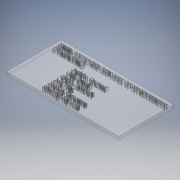
# Autodesk Inventor part: Group Name Plate
Saved by Autodesk Inventor 2018 (Build 220112000, 112)
## iProperties
Created: 2018-11-06
Part Number: Group Name Plate
Material: Generic
Document SubType Name: Modeling
Designer: P300023
Density: 1 g/cm^3
Appearance: Polycarbonate - Clear
Author: P300023
Autodesk Inventor part; units mm, degrees
(part 1 of 4)
ref_plane "YZ Plane" through (0, 0, 0) normal (1, 0, 0) x (0, 1, 0)
ref_plane "XZ Plane" through (0, 0, 0) normal (0, 1, 0) x (-1, 0, 0)
ref_plane "XY Plane" through (0, 0, 0) normal (0, 0, 1) x (1, 0, 0)
sketch "Sketch1" plane through (0, 0, 0) normal (0, 0, 1) x (1, 0, 0)
  line L0 (0, 0) -> (-100, 0)
  line L1 (-100, 0) -> (-100, -49.027)
  line L2 (-100, -49.027) -> (0, -49.027)
  line L3 (0, -49.027) -> (0, 0)
  dimension "d0" = 100
  dimension "d1" = 49.027
  constraints: 8 end point, 2 parallel, 1 horizontal, 1 perpendicular
  measures "d0" distance of L2.end L1.end
  measures "d1" distance of L1.end L0.end
extrude "Extrusion1" add sketch "Sketch1" along normal blind 3
sketch "Sketch2" plane through (0, 0, 3) normal (0, 0, 1) x (1, 0, 0)
  line L0 (-72.5, -15.3818) -> (-27.5, -15.3818) construction
  line L1 (-27.5, -15.3818) -> (-27.5, -49.5595) construction
  line L2 (-27.5, -49.5595) -> (-72.5, -49.5595) construction
  line L3 (-72.5, -49.5595) -> (-72.5, -15.3818) construction
  line L4 (0, 0) -> (-100, 0) projected
  line L5 (-100, -49.027) -> (0, -49.027) projected
  line L6 (0, -49.027) -> (0, 0) projected
  line L7 (-97.5, -2.505) -> (-2.5, -2.505) construction
  line L8 (-2.5, -2.505) -> (-2.5, -5.8685) construction
  line L9 (-2.5, -5.8685) -> (-97.5, -5.8685) construction
  line L10 (-97.5, -5.8685) -> (-97.5, -2.505) construction
  line L11 (-100, 0) -> (-100, -49.027) projected
  spline S0 degree 2 poles (-70.97, -17.892) (-70.97, -18.3121) (-71.4835, -18.7685) (-71.9165, -18.7685) knots 0 0 0 1 2 2 2
  spline S1 degree 2 poles (-71.9165, -18.7685) (-72.0203, -18.7685) (-72.3652, -18.7322) (-72.4818, -18.7063) knots 0 0 0 1 2 2 2
  line L12 (-72.4818, -18.7063) -> (-72.4818, -18.2966)
  line L13 (-72.4818, -18.2966) -> (-72.4585, -18.2966)
  spline S2 degree 2 poles (-72.4585, -18.2966) (-72.3703, -18.3277) (-72.1084, -18.4003) (-71.9736, -18.4003) knots 0 0 0 1 2 2 2
  spline S3 degree 2 poles (-71.9736, -18.4003) (-71.7765, -18.4003) (-71.5405, -18.3096) (-71.4861, -18.2266) knots 0 0 0 1 2 2 2
  spline S4 degree 2 poles (-71.4861, -18.2266) (-71.4264, -18.141) (-71.3953, -17.892) (-71.3953, -17.7287) knots 0 0 0 1 2 2 2
  line L14 (-71.3953, -17.7287) -> (-71.3953, -15.8642)
  line L15 (-71.3953, -15.8642) -> (-72.0721, -15.8642)
  line L16 (-72.0721, -15.8642) -> (-72.0721, -15.5245)
  line L17 (-72.0721, -15.5245) -> (-70.97, -15.5245)
  line L18 (-70.97, -15.5245) -> (-70.97, -17.892)
  spline S5 degree 2 poles (-69.3311, -18.7789) (-69.9068, -18.7789) (-70.5395, -18.1332) (-70.5395, -17.5368) knots 0 0 0 1 2 2 2
  spline S6 degree 2 poles (-70.5395, -17.5368) (-70.5395, -16.9507) (-69.925, -16.2557) (-69.4297, -16.2557) knots 0 0 0 1 2 2 2
  spline S7 degree 2 poles (-69.4297, -16.2557) (-69.2066, -16.2557) (-68.8618, -16.3854) (-68.7347, -16.5228) knots 0 0 0 1 2 2 2
  spline S8 degree 2 poles (-68.7347, -16.5228) (-68.605, -16.6603) (-68.4676, -17.057) (-68.4676, -17.3449) knots 0 0 0 1 2 2 2
  line L19 (-68.4676, -17.3449) -> (-68.4676, -17.5653)
  line L20 (-68.4676, -17.5653) -> (-70.1298, -17.5653)
  spline S9 degree 2 poles (-70.1298, -17.5653) (-70.1298, -17.9828) (-69.7097, -18.4262) (-69.3363, -18.4262) knots 0 0 0 1 2 2 2
  spline S10 degree 2 poles (-69.3363, -18.4262) (-69.2041, -18.4262) (-68.9473, -18.3666) (-68.8436, -18.3199) knots 0 0 0 1 2 2 2
  spline S11 degree 2 poles (-68.8436, -18.3199) (-68.7347, -18.2681) (-68.5843, -18.1773) (-68.535, -18.1358) knots 0 0 0 1 2 2 2
  line L21 (-68.535, -18.1358) -> (-68.5117, -18.1358)
  line L22 (-68.5117, -18.1358) -> (-68.5117, -18.5767)
  spline S12 degree 2 poles (-68.5117, -18.5767) (-68.5817, -18.6052) (-68.7943, -18.6882) (-68.8773, -18.7115) knots 0 0 0 1 2 2 2
  spline S13 degree 2 poles (-68.8773, -18.7115) (-68.994, -18.7452) (-69.1859, -18.7789) (-69.3311, -18.7789) knots 0 0 0 1 2 2 2
  spline S14 degree 2 poles (-68.8618, -17.2567) (-68.8669, -17.0933) (-68.9344, -16.8548) (-68.9992, -16.7744) knots 0 0 0 1 2 2 2
  spline S15 degree 2 poles (-68.9992, -16.7744) (-69.0692, -16.6836) (-69.2896, -16.5877) (-69.453, -16.5877) knots 0 0 0 1 2 2 2
  spline S16 degree 2 poles (-69.453, -16.5877) (-69.6138, -16.5877) (-69.8394, -16.6836) (-69.9327, -16.777) knots 0 0 0 1 2 2 2
  spline S17 degree 2 poles (-69.9327, -16.777) (-70.0235, -16.8729) (-70.1169, -17.1037) (-70.1298, -17.2567) knots 0 0 0 1 2 2 2
  line L23 (-70.1298, -17.2567) -> (-68.8618, -17.2567)
  line L24 (-66.7846, -16.7562) -> (-66.8053, -16.7562)
  spline S18 degree 2 poles (-66.8053, -16.7562) (-66.852, -16.7433) (-66.9532, -16.7381) (-67.0232, -16.7381) knots 0 0 0 1 2 2 2
  spline S19 degree 2 poles (-67.0232, -16.7381) (-67.1865, -16.7381) (-67.5081, -16.8807) (-67.6533, -17.0207) knots 0 0 0 1 2 2 2
  line L25 (-67.6533, -17.0207) -> (-67.6533, -18.7245)
  line L26 (-67.6533, -18.7245) -> (-68.0579, -18.7245)
  line L27 (-68.0579, -18.7245) -> (-68.0579, -16.3232)
  line L28 (-68.0579, -16.3232) -> (-67.6533, -16.3232)
  line L29 (-67.6533, -16.3232) -> (-67.6533, -16.681)
  spline S20 degree 2 poles (-67.6533, -16.681) (-67.4329, -16.4839) (-67.1036, -16.3232) (-66.948, -16.3232) knots 0 0 0 1 2 2 2
  spline S21 degree 2 poles (-66.948, -16.3232) (-66.8857, -16.3232) (-66.8235, -16.3284) (-66.7846, -16.3361) knots 0 0 0 1 2 2 2
  line L30 (-66.7846, -16.3361) -> (-66.7846, -16.7562)
  line L31 (-66.0585, -18.7245) -> (-66.463, -18.7245)
  line L32 (-66.463, -18.7245) -> (-66.463, -16.3232)
  line L33 (-66.463, -16.3232) -> (-66.0585, -16.3232)
  line L34 (-66.0585, -16.3232) -> (-66.0585, -18.7245)
  line L35 (-66.03, -15.9238) -> (-66.489, -15.9238)
  line L36 (-66.489, -15.9238) -> (-66.489, -15.5037)
  line L37 (-66.489, -15.5037) -> (-66.03, -15.5037)
  line L38 (-66.03, -15.5037) -> (-66.03, -15.9238)
  spline S22 degree 2 poles (-64.5104, -18.7789) (-64.7593, -18.7789) (-65.1716, -18.6259) (-65.3194, -18.4703) knots 0 0 0 1 2 2 2
  spline S23 degree 2 poles (-65.3194, -18.4703) (-65.4673, -18.3173) (-65.6306, -17.8454) (-65.6306, -17.529) knots 0 0 0 1 2 2 2
  spline S24 degree 2 poles (-65.6306, -17.529) (-65.6306, -17.2126) (-65.4621, -16.751) (-65.3194, -16.5955) knots 0 0 0 1 2 2 2
  spline S25 degree 2 poles (-65.3194, -16.5955) (-65.1768, -16.4373) (-64.7541, -16.2687) (-64.5104, -16.2687) knots 0 0 0 1 2 2 2
  spline S26 degree 2 poles (-64.5104, -16.2687) (-64.3133, -16.2687) (-63.9451, -16.3802) (-63.8024, -16.4528) knots 0 0 0 1 2 2 2
  line L39 (-63.8024, -16.4528) -> (-63.8024, -16.9066)
  line L40 (-63.8024, -16.9066) -> (-63.8258, -16.9066)
  spline S27 degree 2 poles (-63.8258, -16.9066) (-63.8699, -16.8703) (-64.0047, -16.777) (-64.1006, -16.7277) knots 0 0 0 1 2 2 2
  spline S28 degree 2 poles (-64.1006, -16.7277) (-64.1862, -16.6862) (-64.4144, -16.6214) (-64.5182, -16.6214) knots 0 0 0 1 2 2 2
  spline S29 degree 2 poles (-64.5182, -16.6214) (-64.8319, -16.6214) (-65.2131, -17.0959) (-65.2131, -17.529) knots 0 0 0 1 2 2 2
  spline S30 degree 2 poles (-65.2131, -17.529) (-65.2131, -17.9517) (-64.8449, -18.4262) (-64.5182, -18.4262) knots 0 0 0 1 2 2 2
  spline S31 degree 2 poles (-64.5182, -18.4262) (-64.3211, -18.4262) (-63.9632, -18.2629) (-63.8258, -18.1358) knots 0 0 0 1 2 2 2
  line L41 (-63.8258, -18.1358) -> (-63.8024, -18.1358)
  line L42 (-63.8024, -18.1358) -> (-63.8024, -18.5896)
  spline S32 degree 2 poles (-63.8024, -18.5896) (-63.8621, -18.6181) (-64.0436, -18.6985) (-64.1162, -18.7167) knots 0 0 0 1 2 2 2
  spline S33 degree 2 poles (-64.1162, -18.7167) (-64.2199, -18.7478) (-64.3833, -18.7789) (-64.5104, -18.7789) knots 0 0 0 1 2 2 2
  line L43 (-61.5489, -18.7245) -> (-61.9535, -18.7245)
  line L44 (-61.9535, -18.7245) -> (-61.9535, -17.3553)
  spline S34 degree 2 poles (-61.9535, -17.3553) (-61.9535, -17.1893) (-61.9846, -16.904) (-62.0313, -16.8185) knots 0 0 0 1 2 2 2
  spline S35 degree 2 poles (-62.0313, -16.8185) (-62.0806, -16.7277) (-62.2569, -16.6395) (-62.4073, -16.6395) knots 0 0 0 1 2 2 2
  spline S36 degree 2 poles (-62.4073, -16.6395) (-62.5577, -16.6395) (-62.8767, -16.8003) (-63.0297, -16.93) knots 0 0 0 1 2 2 2
  line L45 (-63.0297, -16.93) -> (-63.0297, -18.7245)
  line L46 (-63.0297, -18.7245) -> (-63.4342, -18.7245)
  line L47 (-63.4342, -18.7245) -> (-63.4342, -15.3818)
  line L48 (-63.4342, -15.3818) -> (-63.0297, -15.3818)
  line L49 (-63.0297, -15.3818) -> (-63.0297, -16.5903)
  spline S37 degree 2 poles (-63.0297, -16.5903) (-62.8481, -16.4269) (-62.4981, -16.2557) (-62.301, -16.2557) knots 0 0 0 1 2 2 2
  spline S38 degree 2 poles (-62.301, -16.2557) (-61.9483, -16.2557) (-61.5489, -16.7225) (-61.5489, -17.166) knots 0 0 0 1 2 2 2
  line L50 (-61.5489, -17.166) -> (-61.5489, -18.7245)
  spline S39 degree 2 poles (-59.0076, -17.5238) (-59.0076, -18.1306) (-59.5911, -18.7919) (-60.0786, -18.7919) knots 0 0 0 1 2 2 2
  spline S40 degree 2 poles (-60.0786, -18.7919) (-60.5791, -18.7919) (-61.1522, -18.1099) (-61.1522, -17.5238) knots 0 0 0 1 2 2 2
  spline S41 degree 2 poles (-61.1522, -17.5238) (-61.1522, -16.9222) (-60.5609, -16.2557) (-60.0786, -16.2557) knots 0 0 0 1 2 2 2
  spline S42 degree 2 poles (-60.0786, -16.2557) (-59.5911, -16.2557) (-59.0076, -16.9196) (-59.0076, -17.5238) knots 0 0 0 1 2 2 2
  spline S43 degree 2 poles (-59.4251, -17.5238) (-59.4251, -17.057) (-59.7648, -16.6032) (-60.0786, -16.6032) knots 0 0 0 1 2 2 2
  spline S44 degree 2 poles (-60.0786, -16.6032) (-60.3924, -16.6032) (-60.7347, -17.057) (-60.7347, -17.5238) knots 0 0 0 1 2 2 2
  spline S45 degree 2 poles (-60.7347, -17.5238) (-60.7347, -17.9776) (-60.3924, -18.4444) (-60.0786, -18.4444) knots 0 0 0 1 2 2 2
  spline S46 degree 2 poles (-60.0786, -18.4444) (-59.7674, -18.4444) (-59.4251, -17.9854) (-59.4251, -17.5238) knots 0 0 0 1 2 2 2
  spline S47 degree 2 poles (-55.9373, -18.7815) (-56.2485, -18.7815) (-56.7749, -18.5715) (-56.9668, -18.3614) knots 0 0 0 1 2 2 2
  spline S48 degree 2 poles (-56.9668, -18.3614) (-57.1587, -18.154) (-57.3687, -17.5316) (-57.3687, -17.1271) knots 0 0 0 1 2 2 2
  spline S49 degree 2 poles (-57.3687, -17.1271) (-57.3687, -16.7251) (-57.1639, -16.1287) (-56.9694, -15.9083) knots 0 0 0 1 2 2 2
  spline S50 degree 2 poles (-56.9694, -15.9083) (-56.7775, -15.693) (-56.2536, -15.4674) (-55.9295, -15.4674) knots 0 0 0 1 2 2 2
  spline S51 degree 2 poles (-55.9295, -15.4674) (-55.7687, -15.4674) (-55.4861, -15.5141) (-55.3668, -15.5504) knots 0 0 0 1 2 2 2
  spline S52 degree 2 poles (-55.3668, -15.5504) (-55.263, -15.5841) (-55.0478, -15.6801) (-54.9415, -15.7371) knots 0 0 0 1 2 2 2
  line L51 (-54.9415, -15.7371) -> (-54.9415, -16.2506)
  line L52 (-54.9415, -16.2506) -> (-54.9752, -16.2506)
  spline S53 degree 2 poles (-54.9752, -16.2506) (-55.0323, -16.1987) (-55.2086, -16.0535) (-55.3357, -15.9835) knots 0 0 0 1 2 2 2
  spline S54 degree 2 poles (-55.3357, -15.9835) (-55.4575, -15.916) (-55.7454, -15.8305) (-55.9321, -15.8305) knots 0 0 0 1 2 2 2
  spline S55 degree 2 poles (-55.9321, -15.8305) (-56.137, -15.8305) (-56.5026, -15.999) (-56.64, -16.1598) knots 0 0 0 1 2 2 2
  spline S56 degree 2 poles (-56.64, -16.1598) (-56.7749, -16.3232) (-56.9253, -16.8185) (-56.9253, -17.1271) knots 0 0 0 1 2 2 2
  spline S57 degree 2 poles (-56.9253, -17.1271) (-56.9253, -17.4564) (-56.7671, -17.9309) (-56.6297, -18.0943) knots 0 0 0 1 2 2 2
  spline S58 degree 2 poles (-56.6297, -18.0943) (-56.4948, -18.2525) (-56.1344, -18.4133) (-55.9321, -18.4133) knots 0 0 0 1 2 2 2
  spline S59 degree 2 poles (-55.9321, -18.4133) (-55.748, -18.4133) (-55.4342, -18.3225) (-55.3123, -18.2551) knots 0 0 0 1 2 2 2
  spline S60 degree 2 poles (-55.3123, -18.2551) (-55.1956, -18.1877) (-55.0219, -18.0476) (-54.9726, -17.9984) knots 0 0 0 1 2 2 2
  line L53 (-54.9726, -17.9984) -> (-54.9415, -17.9984)
  line L54 (-54.9415, -17.9984) -> (-54.9415, -18.5066)
  spline S61 degree 2 poles (-54.9415, -18.5066) (-55.0478, -18.5559) (-55.2345, -18.6467) (-55.3668, -18.6882) knots 0 0 0 1 2 2 2
  spline S62 degree 2 poles (-55.3668, -18.6882) (-55.5068, -18.7348) (-55.7454, -18.7815) (-55.9373, -18.7815) knots 0 0 0 1 2 2 2
  spline S63 degree 2 poles (-52.6024, -17.5238) (-52.6024, -18.1306) (-53.1859, -18.7919) (-53.6734, -18.7919) knots 0 0 0 1 2 2 2
  spline S64 degree 2 poles (-53.6734, -18.7919) (-54.1739, -18.7919) (-54.747, -18.1099) (-54.747, -17.5238) knots 0 0 0 1 2 2 2
  spline S65 degree 2 poles (-54.747, -17.5238) (-54.747, -16.9222) (-54.1558, -16.2557) (-53.6734, -16.2557) knots 0 0 0 1 2 2 2
  spline S66 degree 2 poles (-53.6734, -16.2557) (-53.1859, -16.2557) (-52.6024, -16.9196) (-52.6024, -17.5238) knots 0 0 0 1 2 2 2
  spline S67 degree 2 poles (-53.0199, -17.5238) (-53.0199, -17.057) (-53.3596, -16.6032) (-53.6734, -16.6032) knots 0 0 0 1 2 2 2
  spline S68 degree 2 poles (-53.6734, -16.6032) (-53.9872, -16.6032) (-54.3295, -17.057) (-54.3295, -17.5238) knots 0 0 0 1 2 2 2
  spline S69 degree 2 poles (-54.3295, -17.5238) (-54.3295, -17.9776) (-53.9872, -18.4444) (-53.6734, -18.4444) knots 0 0 0 1 2 2 2
  spline S70 degree 2 poles (-53.6734, -18.4444) (-53.3622, -18.4444) (-53.0199, -17.9854) (-53.0199, -17.5238) knots 0 0 0 1 2 2 2
  line L55 (-50.3204, -18.7245) -> (-50.725, -18.7245)
  line L56 (-50.725, -18.7245) -> (-50.725, -18.46)
  spline S71 degree 2 poles (-50.725, -18.46) (-50.9117, -18.6233) (-51.2462, -18.7919) (-51.4536, -18.7919) knots 0 0 0 1 2 2 2
  spline S72 degree 2 poles (-51.4536, -18.7919) (-51.6092, -18.7919) (-51.8867, -18.6882) (-51.9878, -18.5767) knots 0 0 0 1 2 2 2
  spline S73 degree 2 poles (-51.9878, -18.5767) (-52.0916, -18.4651) (-52.2057, -18.1254) (-52.2057, -17.8817) knots 0 0 0 1 2 2 2
  line L57 (-52.2057, -17.8817) -> (-52.2057, -16.3232)
  line L58 (-52.2057, -16.3232) -> (-51.8011, -16.3232)
  line L59 (-51.8011, -16.3232) -> (-51.8011, -17.6924)
  spline S74 degree 2 poles (-51.8011, -17.6924) (-51.8011, -17.8843) (-51.7726, -18.1358) (-51.7233, -18.2292) knots 0 0 0 1 2 2 2
  spline S75 degree 2 poles (-51.7233, -18.2292) (-51.6741, -18.3225) (-51.5055, -18.4081) (-51.3473, -18.4081) knots 0 0 0 1 2 2 2
  spline S76 degree 2 poles (-51.3473, -18.4081) (-51.1995, -18.4081) (-50.865, -18.2395) (-50.725, -18.1177) knots 0 0 0 1 2 2 2
  line L60 (-50.725, -18.1177) -> (-50.725, -16.3232)
  line L61 (-50.725, -16.3232) -> (-50.3204, -16.3232)
  line L62 (-50.3204, -16.3232) -> (-50.3204, -18.7245)
  line L63 (-47.8491, -18.7245) -> (-48.2536, -18.7245)
  line L64 (-48.2536, -18.7245) -> (-48.2536, -17.3553)
  spline S77 degree 2 poles (-48.2536, -17.3553) (-48.2536, -17.1893) (-48.2848, -16.904) (-48.3314, -16.8185) knots 0 0 0 1 2 2 2
  spline S78 degree 2 poles (-48.3314, -16.8185) (-48.3807, -16.7277) (-48.5571, -16.6395) (-48.7075, -16.6395) knots 0 0 0 1 2 2 2
  spline S79 degree 2 poles (-48.7075, -16.6395) (-48.8579, -16.6395) (-49.1768, -16.8003) (-49.3298, -16.93) knots 0 0 0 1 2 2 2
  line L65 (-49.3298, -16.93) -> (-49.3298, -18.7245)
  line L66 (-49.3298, -18.7245) -> (-49.7344, -18.7245)
  line L67 (-49.7344, -18.7245) -> (-49.7344, -16.3232)
  line L68 (-49.7344, -16.3232) -> (-49.3298, -16.3232)
  line L69 (-49.3298, -16.3232) -> (-49.3298, -16.5903)
  spline S80 degree 2 poles (-49.3298, -16.5903) (-49.1483, -16.4269) (-48.7982, -16.2557) (-48.6011, -16.2557) knots 0 0 0 1 2 2 2
  spline S81 degree 2 poles (-48.6011, -16.2557) (-48.2485, -16.2557) (-47.8491, -16.7225) (-47.8491, -17.166) knots 0 0 0 1 2 2 2
  line L70 (-47.8491, -17.166) -> (-47.8491, -18.7245)
  spline S82 degree 2 poles (-46.6329, -18.7815) (-46.8741, -18.7815) (-47.2916, -18.6519) (-47.429, -18.5792) knots 0 0 0 1 2 2 2
  line L71 (-47.429, -18.5792) -> (-47.429, -18.1254)
  line L72 (-47.429, -18.1254) -> (-47.4083, -18.1254)
  spline S83 degree 2 poles (-47.4083, -18.1254) (-47.3564, -18.1669) (-47.2164, -18.2655) (-47.0997, -18.3199) knots 0 0 0 1 2 2 2
  spline S84 degree 2 poles (-47.0997, -18.3199) (-46.9985, -18.3692) (-46.7496, -18.4418) (-46.6173, -18.4418) knots 0 0 0 1 2 2 2
  spline S85 degree 2 poles (-46.6173, -18.4418) (-46.5214, -18.4418) (-46.301, -18.3977) (-46.2491, -18.3614) knots 0 0 0 1 2 2 2
  spline S86 degree 2 poles (-46.2491, -18.3614) (-46.1739, -18.3121) (-46.1065, -18.2006) (-46.1065, -18.0865) knots 0 0 0 1 2 2 2
  spline S87 degree 2 poles (-46.1065, -18.0865) (-46.1065, -17.9439) (-46.2621, -17.7961) (-46.4618, -17.7468) knots 0 0 0 1 2 2 2
  spline S88 degree 2 poles (-46.4618, -17.7468) (-46.5395, -17.7287) (-46.7885, -17.6768) (-46.8948, -17.6483) knots 0 0 0 1 2 2 2
  spline S89 degree 2 poles (-46.8948, -17.6483) (-47.1697, -17.5679) (-47.4186, -17.236) (-47.4186, -17) knots 0 0 0 1 2 2 2
  spline S90 degree 2 poles (-47.4186, -17) (-47.4186, -16.6732) (-46.9285, -16.2661) (-46.524, -16.2661) knots 0 0 0 1 2 2 2
  spline S91 degree 2 poles (-46.524, -16.2661) (-46.3243, -16.2661) (-45.9198, -16.3647) (-45.7823, -16.4399) knots 0 0 0 1 2 2 2
  line L73 (-45.7823, -16.4399) -> (-45.7823, -16.8729)
  line L74 (-45.7823, -16.8729) -> (-45.8031, -16.8729)
  spline S92 degree 2 poles (-45.8031, -16.8729) (-45.9587, -16.7485) (-46.3373, -16.6058) (-46.5318, -16.6058) knots 0 0 0 1 2 2 2
  spline S93 degree 2 poles (-46.5318, -16.6058) (-46.7314, -16.6058) (-47.0063, -16.7744) (-47.0063, -16.9429) knots 0 0 0 1 2 2 2
  spline S94 degree 2 poles (-47.0063, -16.9429) (-47.0063, -17.0959) (-46.843, -17.2438) (-46.6614, -17.2904) knots 0 0 0 1 2 2 2
  spline S95 degree 2 poles (-46.6614, -17.2904) (-46.5733, -17.3138) (-46.3502, -17.3604) (-46.2284, -17.389) knots 0 0 0 1 2 2 2
  spline S96 degree 2 poles (-46.2284, -17.389) (-45.9639, -17.4564) (-45.6942, -17.765) (-45.6942, -18.0321) knots 0 0 0 1 2 2 2
  spline S97 degree 2 poles (-45.6942, -18.0321) (-45.6942, -18.1877) (-45.816, -18.4626) (-45.9353, -18.5637) knots 0 0 0 1 2 2 2
  spline S98 degree 2 poles (-45.9353, -18.5637) (-46.0624, -18.67) (-46.3865, -18.7815) (-46.6329, -18.7815) knots 0 0 0 1 2 2 2
  spline S99 degree 2 poles (-44.2757, -18.7789) (-44.8514, -18.7789) (-45.4841, -18.1332) (-45.4841, -17.5368) knots 0 0 0 1 2 2 2
  spline S100 degree 2 poles (-45.4841, -17.5368) (-45.4841, -16.9507) (-44.8695, -16.2557) (-44.3742, -16.2557) knots 0 0 0 1 2 2 2
  spline S101 degree 2 poles (-44.3742, -16.2557) (-44.1512, -16.2557) (-43.8063, -16.3854) (-43.6793, -16.5228) knots 0 0 0 1 2 2 2
  spline S102 degree 2 poles (-43.6793, -16.5228) (-43.5496, -16.6603) (-43.4122, -17.057) (-43.4122, -17.3449) knots 0 0 0 1 2 2 2
  line L75 (-43.4122, -17.3449) -> (-43.4122, -17.5653)
  line L76 (-43.4122, -17.5653) -> (-45.0744, -17.5653)
  spline S103 degree 2 poles (-45.0744, -17.5653) (-45.0744, -17.9828) (-44.6543, -18.4262) (-44.2809, -18.4262) knots 0 0 0 1 2 2 2
  spline S104 degree 2 poles (-44.2809, -18.4262) (-44.1486, -18.4262) (-43.8919, -18.3666) (-43.7882, -18.3199) knots 0 0 0 1 2 2 2
  spline S105 degree 2 poles (-43.7882, -18.3199) (-43.6793, -18.2681) (-43.5288, -18.1773) (-43.4796, -18.1358) knots 0 0 0 1 2 2 2
  line L77 (-43.4796, -18.1358) -> (-43.4562, -18.1358)
  line L78 (-43.4562, -18.1358) -> (-43.4562, -18.5767)
  spline S106 degree 2 poles (-43.4562, -18.5767) (-43.5263, -18.6052) (-43.7389, -18.6882) (-43.8219, -18.7115) knots 0 0 0 1 2 2 2
  spline S107 degree 2 poles (-43.8219, -18.7115) (-43.9386, -18.7452) (-44.1305, -18.7789) (-44.2757, -18.7789) knots 0 0 0 1 2 2 2
  spline S108 degree 2 poles (-43.8063, -17.2567) (-43.8115, -17.0933) (-43.8789, -16.8548) (-43.9438, -16.7744) knots 0 0 0 1 2 2 2
  spline S109 degree 2 poles (-43.9438, -16.7744) (-44.0138, -16.6836) (-44.2342, -16.5877) (-44.3976, -16.5877) knots 0 0 0 1 2 2 2
  spline S110 degree 2 poles (-44.3976, -16.5877) (-44.5583, -16.5877) (-44.784, -16.6836) (-44.8773, -16.777) knots 0 0 0 1 2 2 2
  spline S111 degree 2 poles (-44.8773, -16.777) (-44.9681, -16.8729) (-45.0614, -17.1037) (-45.0744, -17.2567) knots 0 0 0 1 2 2 2
  line L79 (-45.0744, -17.2567) -> (-43.8063, -17.2567)
  line L80 (-42.5901, -18.7245) -> (-42.9947, -18.7245)
  line L81 (-42.9947, -18.7245) -> (-42.9947, -15.3818)
  line L82 (-42.9947, -15.3818) -> (-42.5901, -15.3818)
  line L83 (-42.5901, -15.3818) -> (-42.5901, -18.7245)
  spline S112 degree 2 poles (-69.912, -21.1588) (-69.7305, -21.3715) (-69.5282, -21.9938) (-69.5282, -22.3932) knots 0 0 0 1 2 2 2
  spline S113 degree 2 poles (-69.5282, -22.3932) (-69.5282, -22.7822) (-69.7253, -23.4123) (-69.912, -23.6249) knots 0 0 0 1 2 2 2
  spline S114 degree 2 poles (-69.912, -23.6249) (-70.1091, -23.848) (-70.6303, -24.0606) (-70.9441, -24.0606) knots 0 0 0 1 2 2 2
  spline S115 degree 2 poles (-70.9441, -24.0606) (-71.2682, -24.0606) (-71.7869, -23.8402) (-71.9762, -23.6249) knots 0 0 0 1 2 2 2
  spline S116 degree 2 poles (-71.9762, -23.6249) (-72.1603, -23.4123) (-72.3574, -22.7873) (-72.3574, -22.3932) knots 0 0 0 1 2 2 2
  spline S117 degree 2 poles (-72.3574, -22.3932) (-72.3574, -21.9912) (-72.1577, -21.3792) (-71.9736, -21.1588) knots 0 0 0 1 2 2 2
  spline S118 degree 2 poles (-71.9736, -21.1588) (-71.7869, -20.9462) (-71.2656, -20.7258) (-70.9441, -20.7258) knots 0 0 0 1 2 2 2
  spline S119 degree 2 poles (-70.9441, -20.7258) (-70.6173, -20.7258) (-70.0935, -20.954) (-69.912, -21.1588) knots 0 0 0 1 2 2 2
  spline S120 degree 2 poles (-69.9716, -22.3932) (-69.9716, -22.0768) (-70.1091, -21.5867) (-70.2335, -21.4259) knots 0 0 0 1 2 2 2
  spline S121 degree 2 poles (-70.2335, -21.4259) (-70.3606, -21.26) (-70.7185, -21.094) (-70.9415, -21.094) knots 0 0 0 1 2 2 2
  spline S122 degree 2 poles (-70.9415, -21.094) (-71.1723, -21.094) (-71.5198, -21.2548) (-71.652, -21.4259) knots 0 0 0 1 2 2 2
  spline S123 degree 2 poles (-71.652, -21.4259) (-71.7791, -21.5893) (-71.9139, -22.082) (-71.9139, -22.3932) knots 0 0 0 1 2 2 2
  spline S124 degree 2 poles (-71.9139, -22.3932) (-71.9139, -23.0233) (-71.3849, -23.6924) (-70.9415, -23.6924) knots 0 0 0 1 2 2 2
  spline S125 degree 2 poles (-70.9415, -23.6924) (-70.4981, -23.6924) (-69.9716, -23.0233) (-69.9716, -22.3932) knots 0 0 0 1 2 2 2
  spline S126 degree 2 poles (-68.3665, -24.0399) (-68.6958, -24.0399) (-69.0666, -23.6638) (-69.0666, -23.2567) knots 0 0 0 1 2 2 2
  line L84 (-69.0666, -23.2567) -> (-69.0666, -21.9264)
  line L85 (-69.0666, -21.9264) -> (-69.3389, -21.9264)
  line L86 (-69.3389, -21.9264) -> (-69.3389, -21.5919)
  line L87 (-69.3389, -21.5919) -> (-69.0666, -21.5919)
  line L88 (-69.0666, -21.5919) -> (-69.0666, -20.9021)
  line L89 (-69.0666, -20.9021) -> (-68.6621, -20.9021)
  line L90 (-68.6621, -20.9021) -> (-68.6621, -21.5919)
  line L91 (-68.6621, -21.5919) -> (-67.9178, -21.5919)
  line L92 (-67.9178, -21.5919) -> (-67.9178, -21.9264)
  line L93 (-67.9178, -21.9264) -> (-68.6621, -21.9264)
  line L94 (-68.6621, -21.9264) -> (-68.6621, -23.07)
  spline S127 degree 2 poles (-68.6621, -23.07) (-68.6621, -23.2515) (-68.6491, -23.4512) (-68.605, -23.5368) knots 0 0 0 1 2 2 2
  spline S128 degree 2 poles (-68.605, -23.5368) (-68.5687, -23.612) (-68.4053, -23.6872) (-68.2653, -23.6872) knots 0 0 0 1 2 2 2
  spline S129 degree 2 poles (-68.2653, -23.6872) (-68.1668, -23.6872) (-67.9827, -23.6275) (-67.9412, -23.6094) knots 0 0 0 1 2 2 2
  line L95 (-67.9412, -23.6094) -> (-67.9178, -23.6094)
  line L96 (-67.9178, -23.6094) -> (-67.9178, -23.9724)
  spline S130 degree 2 poles (-67.9178, -23.9724) (-68.0319, -24.0036) (-68.2653, -24.0399) (-68.3665, -24.0399) knots 0 0 0 1 2 2 2
  line L97 (-67.2073, -23.9932) -> (-67.6118, -23.9932)
  line L98 (-67.6118, -23.9932) -> (-67.6118, -21.5919)
  line L99 (-67.6118, -21.5919) -> (-67.2073, -21.5919)
  line L100 (-67.2073, -21.5919) -> (-67.2073, -23.9932)
  line L101 (-67.1788, -21.1925) -> (-67.6378, -21.1925)
  line L102 (-67.6378, -21.1925) -> (-67.6378, -20.7724)
  line L103 (-67.6378, -20.7724) -> (-67.1788, -20.7724)
  line L104 (-67.1788, -20.7724) -> (-67.1788, -21.1925)
  spline S131 degree 2 poles (-65.9652, -24.0502) (-66.2063, -24.0502) (-66.6238, -23.9206) (-66.7613, -23.848) knots 0 0 0 1 2 2 2
  line L105 (-66.7613, -23.848) -> (-66.7613, -23.3942)
  line L106 (-66.7613, -23.3942) -> (-66.7405, -23.3942)
  spline S132 degree 2 poles (-66.7405, -23.3942) (-66.6887, -23.4356) (-66.5486, -23.5342) (-66.4319, -23.5886) knots 0 0 0 1 2 2 2
  spline S133 degree 2 poles (-66.4319, -23.5886) (-66.3308, -23.6379) (-66.0818, -23.7105) (-65.9496, -23.7105) knots 0 0 0 1 2 2 2
  spline S134 degree 2 poles (-65.9496, -23.7105) (-65.8536, -23.7105) (-65.6332, -23.6664) (-65.5814, -23.6301) knots 0 0 0 1 2 2 2
  spline S135 degree 2 poles (-65.5814, -23.6301) (-65.5062, -23.5809) (-65.4387, -23.4694) (-65.4387, -23.3553) knots 0 0 0 1 2 2 2
  spline S136 degree 2 poles (-65.4387, -23.3553) (-65.4387, -23.2126) (-65.5943, -23.0648) (-65.794, -23.0155) knots 0 0 0 1 2 2 2
  spline S137 degree 2 poles (-65.794, -23.0155) (-65.8718, -22.9974) (-66.1207, -22.9455) (-66.2271, -22.917) knots 0 0 0 1 2 2 2
  spline S138 degree 2 poles (-66.2271, -22.917) (-66.5019, -22.8366) (-66.7509, -22.5047) (-66.7509, -22.2687) knots 0 0 0 1 2 2 2
  spline S139 degree 2 poles (-66.7509, -22.2687) (-66.7509, -21.942) (-66.2608, -21.5348) (-65.8562, -21.5348) knots 0 0 0 1 2 2 2
  spline S140 degree 2 poles (-65.8562, -21.5348) (-65.6566, -21.5348) (-65.252, -21.6334) (-65.1146, -21.7086) knots 0 0 0 1 2 2 2
  line L107 (-65.1146, -21.7086) -> (-65.1146, -22.1416)
  line L108 (-65.1146, -22.1416) -> (-65.1353, -22.1416)
  spline S141 degree 2 poles (-65.1353, -22.1416) (-65.2909, -22.0172) (-65.6695, -21.8745) (-65.864, -21.8745) knots 0 0 0 1 2 2 2
  spline S142 degree 2 poles (-65.864, -21.8745) (-66.0637, -21.8745) (-66.3386, -22.0431) (-66.3386, -22.2117) knots 0 0 0 1 2 2 2
  spline S143 degree 2 poles (-66.3386, -22.2117) (-66.3386, -22.3647) (-66.1752, -22.5125) (-65.9937, -22.5591) knots 0 0 0 1 2 2 2
  spline S144 degree 2 poles (-65.9937, -22.5591) (-65.9055, -22.5825) (-65.6825, -22.6292) (-65.5606, -22.6577) knots 0 0 0 1 2 2 2
  spline S145 degree 2 poles (-65.5606, -22.6577) (-65.2961, -22.7251) (-65.0264, -23.0337) (-65.0264, -23.3008) knots 0 0 0 1 2 2 2
  spline S146 degree 2 poles (-65.0264, -23.3008) (-65.0264, -23.4564) (-65.1483, -23.7313) (-65.2676, -23.8324) knots 0 0 0 1 2 2 2
  spline S147 degree 2 poles (-65.2676, -23.8324) (-65.3947, -23.9387) (-65.7188, -24.0502) (-65.9652, -24.0502) knots 0 0 0 1 2 2 2
  spline S148 degree 2 poles (-61.9042, -24.0554) (-62.2439, -24.0554) (-62.8066, -23.848) (-63.0089, -23.6379) knots 0 0 0 1 2 2 2
  spline S149 degree 2 poles (-63.0089, -23.6379) (-63.2112, -23.4253) (-63.4264, -22.7977) (-63.4264, -22.3906) knots 0 0 0 1 2 2 2
  spline S150 degree 2 poles (-63.4264, -22.3906) (-63.4264, -22.0042) (-63.2086, -21.3922) (-63.0063, -21.1744) knots 0 0 0 1 2 2 2
  spline S151 degree 2 poles (-63.0063, -21.1744) (-62.8118, -20.9643) (-62.2413, -20.7361) (-61.9016, -20.7361) knots 0 0 0 1 2 2 2
  spline S152 degree 2 poles (-61.9016, -20.7361) (-61.7382, -20.7361) (-61.4426, -20.7828) (-61.3078, -20.8243) knots 0 0 0 1 2 2 2
  spline S153 degree 2 poles (-61.3078, -20.8243) (-61.1989, -20.8554) (-60.9344, -20.9695) (-60.854, -21.011) knots 0 0 0 1 2 2 2
  line L109 (-60.854, -21.011) -> (-60.854, -21.5245)
  line L110 (-60.854, -21.5245) -> (-60.8903, -21.5245)
  spline S154 degree 2 poles (-60.8903, -21.5245) (-60.9707, -21.4544) (-61.1392, -21.3274) (-61.2948, -21.2548) knots 0 0 0 1 2 2 2
  spline S155 degree 2 poles (-61.2948, -21.2548) (-61.4245, -21.1899) (-61.759, -21.1044) (-61.9509, -21.1044) knots 0 0 0 1 2 2 2
  spline S156 degree 2 poles (-61.9509, -21.1044) (-62.4125, -21.1044) (-62.983, -21.7993) (-62.983, -22.3776) knots 0 0 0 1 2 2 2
  spline S157 degree 2 poles (-62.983, -22.3776) (-62.983, -22.6992) (-62.8326, -23.1815) (-62.69, -23.3475) knots 0 0 0 1 2 2 2
  spline S158 degree 2 poles (-62.69, -23.3475) (-62.5525, -23.5134) (-62.1635, -23.6872) (-61.9198, -23.6872) knots 0 0 0 1 2 2 2
  spline S159 degree 2 poles (-61.9198, -23.6872) (-61.7408, -23.6872) (-61.383, -23.6353) (-61.2611, -23.5835) knots 0 0 0 1 2 2 2
  line L111 (-61.2611, -23.5835) -> (-61.2611, -22.7562)
  line L112 (-61.2611, -22.7562) -> (-62.0028, -22.7562)
  line L113 (-62.0028, -22.7562) -> (-62.0028, -22.3828)
  line L114 (-62.0028, -22.3828) -> (-60.841, -22.3828)
  line L115 (-60.841, -22.3828) -> (-60.841, -23.7805)
  spline S160 degree 2 poles (-60.841, -23.7805) (-60.9214, -23.8168) (-61.1963, -23.9284) (-61.313, -23.9621) knots 0 0 0 1 2 2 2
  spline S161 degree 2 poles (-61.313, -23.9621) (-61.4712, -24.0087) (-61.7253, -24.0554) (-61.9042, -24.0554) knots 0 0 0 1 2 2 2
  line L116 (-59.0647, -22.0249) -> (-59.0854, -22.0249)
  spline S162 degree 2 poles (-59.0854, -22.0249) (-59.1321, -22.012) (-59.2332, -22.0068) (-59.3032, -22.0068) knots 0 0 0 1 2 2 2
  spline S163 degree 2 poles (-59.3032, -22.0068) (-59.4666, -22.0068) (-59.7882, -22.1494) (-59.9334, -22.2895) knots 0 0 0 1 2 2 2
  line L117 (-59.9334, -22.2895) -> (-59.9334, -23.9932)
  line L118 (-59.9334, -23.9932) -> (-60.3379, -23.9932)
  line L119 (-60.3379, -23.9932) -> (-60.3379, -21.5919)
  line L120 (-60.3379, -21.5919) -> (-59.9334, -21.5919)
  line L121 (-59.9334, -21.5919) -> (-59.9334, -21.9497)
  spline S164 degree 2 poles (-59.9334, -21.9497) (-59.713, -21.7527) (-59.3836, -21.5919) (-59.228, -21.5919) knots 0 0 0 1 2 2 2
  spline S165 degree 2 poles (-59.228, -21.5919) (-59.1658, -21.5919) (-59.1036, -21.5971) (-59.0647, -21.6048) knots 0 0 0 1 2 2 2
  line L122 (-59.0647, -21.6048) -> (-59.0647, -22.0249)
  spline S166 degree 2 poles (-57.4128, -23.739) (-57.4621, -23.7754) (-57.628, -23.905) (-57.7058, -23.9439) knots 0 0 0 1 2 2 2
  spline S167 degree 2 poles (-57.7058, -23.9439) (-57.8122, -24.001) (-58.0118, -24.0606) (-58.1934, -24.0606) knots 0 0 0 1 2 2 2
  spline S168 degree 2 poles (-58.1934, -24.0606) (-58.3412, -24.0606) (-58.6083, -23.9491) (-58.7094, -23.848) knots 0 0 0 1 2 2 2
  spline S169 degree 2 poles (-58.7094, -23.848) (-58.8053, -23.7494) (-58.922, -23.459) (-58.922, -23.2982) knots 0 0 0 1 2 2 2
  spline S170 degree 2 poles (-58.922, -23.2982) (-58.922, -23.0493) (-58.712, -22.6966) (-58.4838, -22.5954) knots 0 0 0 1 2 2 2
  spline S171 degree 2 poles (-58.4838, -22.5954) (-58.2815, -22.5021) (-57.7318, -22.4321) (-57.4128, -22.4139) knots 0 0 0 1 2 2 2
  line L123 (-57.4128, -22.4139) -> (-57.4128, -22.3361)
  spline S172 degree 2 poles (-57.4128, -22.3361) (-57.4128, -22.1961) (-57.4984, -22.0224) (-57.5762, -21.9731) knots 0 0 0 1 2 2 2
  spline S173 degree 2 poles (-57.5762, -21.9731) (-57.654, -21.9238) (-57.877, -21.8927) (-57.9963, -21.8927) knots 0 0 0 1 2 2 2
  spline S174 degree 2 poles (-57.9963, -21.8927) (-58.1363, -21.8927) (-58.5149, -21.9757) (-58.7042, -22.0561) knots 0 0 0 1 2 2 2
  line L124 (-58.7042, -22.0561) -> (-58.7276, -22.0561)
  line L125 (-58.7276, -22.0561) -> (-58.7276, -21.6437)
  spline S175 degree 2 poles (-58.7276, -21.6437) (-58.616, -21.6126) (-58.1985, -21.5348) (-57.9937, -21.5348) knots 0 0 0 1 2 2 2
  spline S176 degree 2 poles (-57.9937, -21.5348) (-57.7447, -21.5348) (-57.405, -21.6126) (-57.2702, -21.7138) knots 0 0 0 1 2 2 2
  spline S177 degree 2 poles (-57.2702, -21.7138) (-57.1379, -21.8123) (-57.0083, -22.1261) (-57.0083, -22.3517) knots 0 0 0 1 2 2 2
  line L126 (-57.0083, -22.3517) -> (-57.0083, -23.9932)
  line L127 (-57.0083, -23.9932) -> (-57.4128, -23.9932)
  line L128 (-57.4128, -23.9932) -> (-57.4128, -23.739)
  line L129 (-57.4128, -23.4019) -> (-57.4128, -22.7355)
  spline S178 degree 2 poles (-57.4128, -22.7355) (-57.558, -22.7484) (-57.9963, -22.7925) (-58.1337, -22.834) knots 0 0 0 1 2 2 2
  spline S179 degree 2 poles (-58.1337, -22.834) (-58.2945, -22.8833) (-58.5045, -23.0882) (-58.5045, -23.2697) knots 0 0 0 1 2 2 2
  spline S180 degree 2 poles (-58.5045, -23.2697) (-58.5045, -23.4771) (-58.2712, -23.6872) (-58.0481, -23.6872) knots 0 0 0 1 2 2 2
  spline S181 degree 2 poles (-58.0481, -23.6872) (-57.8588, -23.6872) (-57.5477, -23.5238) (-57.4128, -23.4019) knots 0 0 0 1 2 2 2
  spline S182 degree 2 poles (-55.3979, -24.0476) (-55.9736, -24.0476) (-56.6063, -23.4019) (-56.6063, -22.8055) knots 0 0 0 1 2 2 2
  spline S183 degree 2 poles (-56.6063, -22.8055) (-56.6063, -22.2194) (-55.9917, -21.5245) (-55.4964, -21.5245) knots 0 0 0 1 2 2 2
  spline S184 degree 2 poles (-55.4964, -21.5245) (-55.2734, -21.5245) (-54.9285, -21.6541) (-54.8015, -21.7916) knots 0 0 0 1 2 2 2
  spline S185 degree 2 poles (-54.8015, -21.7916) (-54.6718, -21.929) (-54.5344, -22.3258) (-54.5344, -22.6136) knots 0 0 0 1 2 2 2
  line L130 (-54.5344, -22.6136) -> (-54.5344, -22.834)
  line L131 (-54.5344, -22.834) -> (-56.1966, -22.834)
  spline S186 degree 2 poles (-56.1966, -22.834) (-56.1966, -23.2515) (-55.7765, -23.695) (-55.4031, -23.695) knots 0 0 0 1 2 2 2
  spline S187 degree 2 poles (-55.4031, -23.695) (-55.2708, -23.695) (-55.0141, -23.6353) (-54.9104, -23.5886) knots 0 0 0 1 2 2 2
  spline S188 degree 2 poles (-54.9104, -23.5886) (-54.8015, -23.5368) (-54.6511, -23.446) (-54.6018, -23.4045) knots 0 0 0 1 2 2 2
  line L132 (-54.6018, -23.4045) -> (-54.5784, -23.4045)
  line L133 (-54.5784, -23.4045) -> (-54.5784, -23.8454)
  spline S189 degree 2 poles (-54.5784, -23.8454) (-54.6485, -23.8739) (-54.8611, -23.9569) (-54.9441, -23.9802) knots 0 0 0 1 2 2 2
  spline S190 degree 2 poles (-54.9441, -23.9802) (-55.0608, -24.0139) (-55.2527, -24.0476) (-55.3979, -24.0476) knots 0 0 0 1 2 2 2
  spline S191 degree 2 poles (-54.9285, -22.5254) (-54.9337, -22.3621) (-55.0011, -22.1235) (-55.066, -22.0431) knots 0 0 0 1 2 2 2
  spline S192 degree 2 poles (-55.066, -22.0431) (-55.136, -21.9523) (-55.3564, -21.8564) (-55.5198, -21.8564) knots 0 0 0 1 2 2 2
  spline S193 degree 2 poles (-55.5198, -21.8564) (-55.6806, -21.8564) (-55.9062, -21.9523) (-55.9995, -22.0457) knots 0 0 0 1 2 2 2
  spline S194 degree 2 poles (-55.9995, -22.0457) (-56.0903, -22.1416) (-56.1836, -22.3724) (-56.1966, -22.5254) knots 0 0 0 1 2 2 2
  line L134 (-56.1966, -22.5254) -> (-54.9285, -22.5254)
  spline S195 degree 2 poles (-53.3985, -24.0399) (-53.7279, -24.0399) (-54.0987, -23.6638) (-54.0987, -23.2567) knots 0 0 0 1 2 2 2
  line L135 (-54.0987, -23.2567) -> (-54.0987, -21.9264)
  line L136 (-54.0987, -21.9264) -> (-54.371, -21.9264)
  line L137 (-54.371, -21.9264) -> (-54.371, -21.5919)
  line L138 (-54.371, -21.5919) -> (-54.0987, -21.5919)
  line L139 (-54.0987, -21.5919) -> (-54.0987, -20.9021)
  line L140 (-54.0987, -20.9021) -> (-53.6942, -20.9021)
  line L141 (-53.6942, -20.9021) -> (-53.6942, -21.5919)
  line L142 (-53.6942, -21.5919) -> (-52.9499, -21.5919)
  line L143 (-52.9499, -21.5919) -> (-52.9499, -21.9264)
  line L144 (-52.9499, -21.9264) -> (-53.6942, -21.9264)
  line L145 (-53.6942, -21.9264) -> (-53.6942, -23.07)
  spline S196 degree 2 poles (-53.6942, -23.07) (-53.6942, -23.2515) (-53.6812, -23.4512) (-53.6371, -23.5368) knots 0 0 0 1 2 2 2
  spline S197 degree 2 poles (-53.6371, -23.5368) (-53.6008, -23.612) (-53.4374, -23.6872) (-53.2974, -23.6872) knots 0 0 0 1 2 2 2
  spline S198 degree 2 poles (-53.2974, -23.6872) (-53.1989, -23.6872) (-53.0147, -23.6275) (-52.9733, -23.6094) knots 0 0 0 1 2 2 2
  line L146 (-52.9733, -23.6094) -> (-52.9499, -23.6094)
  line L147 (-52.9499, -23.6094) -> (-52.9499, -23.9724)
  spline S199 degree 2 poles (-52.9499, -23.9724) (-53.064, -24.0036) (-53.2974, -24.0399) (-53.3985, -24.0399) knots 0 0 0 1 2 2 2
  line L148 (-51.075, -23.9932) -> (-52.8384, -23.9932)
  line L149 (-52.8384, -23.9932) -> (-52.8384, -23.6924)
  line L150 (-52.8384, -23.6924) -> (-51.5833, -21.9238)
  line L151 (-51.5833, -21.9238) -> (-52.7865, -21.9238)
  line L152 (-52.7865, -21.9238) -> (-52.7865, -21.5919)
  line L153 (-52.7865, -21.5919) -> (-51.0984, -21.5919)
  line L154 (-51.0984, -21.5919) -> (-51.0984, -21.8797)
  line L155 (-51.0984, -21.8797) -> (-52.3587, -23.6535)
  line L156 (-52.3587, -23.6535) -> (-51.075, -23.6535)
  line L157 (-51.075, -23.6535) -> (-51.075, -23.9932)
  spline S200 degree 2 poles (-70.8352, -29.3241) (-71.1749, -29.3241) (-71.7376, -29.1167) (-71.9399, -28.9066) knots 0 0 0 1 2 2 2
  spline S201 degree 2 poles (-71.9399, -28.9066) (-72.1421, -28.694) (-72.3574, -28.0664) (-72.3574, -27.6593) knots 0 0 0 1 2 2 2
  spline S202 degree 2 poles (-72.3574, -27.6593) (-72.3574, -27.2729) (-72.1395, -26.6609) (-71.9373, -26.4431) knots 0 0 0 1 2 2 2
  spline S203 degree 2 poles (-71.9373, -26.4431) (-71.7428, -26.233) (-71.1723, -26.0048) (-70.8326, -26.0048) knots 0 0 0 1 2 2 2
  spline S204 degree 2 poles (-70.8326, -26.0048) (-70.6692, -26.0048) (-70.3736, -26.0515) (-70.2387, -26.093) knots 0 0 0 1 2 2 2
  spline S205 degree 2 poles (-70.2387, -26.093) (-70.1298, -26.1241) (-69.8653, -26.2382) (-69.7849, -26.2797) knots 0 0 0 1 2 2 2
  line L158 (-69.7849, -26.2797) -> (-69.7849, -26.7932)
  line L159 (-69.7849, -26.7932) -> (-69.8212, -26.7932)
  spline S206 degree 2 poles (-69.8212, -26.7932) (-69.9016, -26.7232) (-70.0702, -26.5961) (-70.2258, -26.5235) knots 0 0 0 1 2 2 2
  spline S207 degree 2 poles (-70.2258, -26.5235) (-70.3554, -26.4587) (-70.69, -26.3731) (-70.8818, -26.3731) knots 0 0 0 1 2 2 2
  spline S208 degree 2 poles (-70.8818, -26.3731) (-71.3434, -26.3731) (-71.9139, -27.0681) (-71.9139, -27.6463) knots 0 0 0 1 2 2 2
  spline S209 degree 2 poles (-71.9139, -27.6463) (-71.9139, -27.9679) (-71.7635, -28.4502) (-71.6209, -28.6162) knots 0 0 0 1 2 2 2
  spline S210 degree 2 poles (-71.6209, -28.6162) (-71.4835, -28.7822) (-71.0945, -28.9559) (-70.8507, -28.9559) knots 0 0 0 1 2 2 2
  spline S211 degree 2 poles (-70.8507, -28.9559) (-70.6718, -28.9559) (-70.3139, -28.904) (-70.1921, -28.8522) knots 0 0 0 1 2 2 2
  line L160 (-70.1921, -28.8522) -> (-70.1921, -28.0249)
  line L161 (-70.1921, -28.0249) -> (-70.9337, -28.0249)
  line L162 (-70.9337, -28.0249) -> (-70.9337, -27.6515)
  line L163 (-70.9337, -27.6515) -> (-69.772, -27.6515)
  line L164 (-69.772, -27.6515) -> (-69.772, -29.0493)
  spline S212 degree 2 poles (-69.772, -29.0493) (-69.8524, -29.0856) (-70.1272, -29.1971) (-70.2439, -29.2308) knots 0 0 0 1 2 2 2
  spline S213 degree 2 poles (-70.2439, -29.2308) (-70.4021, -29.2775) (-70.6562, -29.3241) (-70.8352, -29.3241) knots 0 0 0 1 2 2 2
  line L165 (-68.8566, -29.2619) -> (-69.2611, -29.2619)
  line L166 (-69.2611, -29.2619) -> (-69.2611, -25.9193)
  line L167 (-69.2611, -25.9193) -> (-68.8566, -25.9193)
  line L168 (-68.8566, -25.9193) -> (-68.8566, -29.2619)
  spline S214 degree 2 poles (-67.2203, -29.3164) (-67.7959, -29.3164) (-68.4287, -28.6706) (-68.4287, -28.0742) knots 0 0 0 1 2 2 2
  spline S215 degree 2 poles (-68.4287, -28.0742) (-68.4287, -27.4882) (-67.8141, -26.7932) (-67.3188, -26.7932) knots 0 0 0 1 2 2 2
  spline S216 degree 2 poles (-67.3188, -26.7932) (-67.0958, -26.7932) (-66.7509, -26.9228) (-66.6238, -27.0603) knots 0 0 0 1 2 2 2
  spline S217 degree 2 poles (-66.6238, -27.0603) (-66.4942, -27.1977) (-66.3567, -27.5945) (-66.3567, -27.8823) knots 0 0 0 1 2 2 2
  line L169 (-66.3567, -27.8823) -> (-66.3567, -28.1027)
  line L170 (-66.3567, -28.1027) -> (-68.019, -28.1027)
  spline S218 degree 2 poles (-68.019, -28.1027) (-68.019, -28.5202) (-67.5989, -28.9637) (-67.2254, -28.9637) knots 0 0 0 1 2 2 2
  spline S219 degree 2 poles (-67.2254, -28.9637) (-67.0932, -28.9637) (-66.8365, -28.904) (-66.7327, -28.8574) knots 0 0 0 1 2 2 2
  spline S220 degree 2 poles (-66.7327, -28.8574) (-66.6238, -28.8055) (-66.4734, -28.7147) (-66.4241, -28.6732) knots 0 0 0 1 2 2 2
  line L171 (-66.4241, -28.6732) -> (-66.4008, -28.6732)
  line L172 (-66.4008, -28.6732) -> (-66.4008, -29.1141)
  spline S221 degree 2 poles (-66.4008, -29.1141) (-66.4708, -29.1426) (-66.6835, -29.2256) (-66.7665, -29.2489) knots 0 0 0 1 2 2 2
  spline S222 degree 2 poles (-66.7665, -29.2489) (-66.8831, -29.2826) (-67.075, -29.3164) (-67.2203, -29.3164) knots 0 0 0 1 2 2 2
  spline S223 degree 2 poles (-66.7509, -27.7941) (-66.7561, -27.6308) (-66.8235, -27.3922) (-66.8883, -27.3118) knots 0 0 0 1 2 2 2
  spline S224 degree 2 poles (-66.8883, -27.3118) (-66.9583, -27.2211) (-67.1788, -27.1251) (-67.3421, -27.1251) knots 0 0 0 1 2 2 2
  spline S225 degree 2 poles (-67.3421, -27.1251) (-67.5029, -27.1251) (-67.7285, -27.2211) (-67.8219, -27.3144) knots 0 0 0 1 2 2 2
  spline S226 degree 2 poles (-67.8219, -27.3144) (-67.9126, -27.4104) (-68.006, -27.6412) (-68.019, -27.7941) knots 0 0 0 1 2 2 2
  line L173 (-68.019, -27.7941) -> (-66.7509, -27.7941)
  line L174 (-64.0618, -29.2619) -> (-64.4663, -29.2619)
  line L175 (-64.4663, -29.2619) -> (-64.4663, -27.8927)
  spline S227 degree 2 poles (-64.4663, -27.8927) (-64.4663, -27.7267) (-64.4974, -27.4415) (-64.5441, -27.3559) knots 0 0 0 1 2 2 2
  spline S228 degree 2 poles (-64.5441, -27.3559) (-64.5934, -27.2651) (-64.7697, -27.177) (-64.9201, -27.177) knots 0 0 0 1 2 2 2
  spline S229 degree 2 poles (-64.9201, -27.177) (-65.0705, -27.177) (-65.3895, -27.3377) (-65.5425, -27.4674) knots 0 0 0 1 2 2 2
  line L176 (-65.5425, -27.4674) -> (-65.5425, -29.2619)
  line L177 (-65.5425, -29.2619) -> (-65.947, -29.2619)
  line L178 (-65.947, -29.2619) -> (-65.947, -26.8606)
  line L179 (-65.947, -26.8606) -> (-65.5425, -26.8606)
  line L180 (-65.5425, -26.8606) -> (-65.5425, -27.1277)
  spline S230 degree 2 poles (-65.5425, -27.1277) (-65.3609, -26.9643) (-65.0109, -26.7932) (-64.8138, -26.7932) knots 0 0 0 1 2 2 2
  spline S231 degree 2 poles (-64.8138, -26.7932) (-64.4611, -26.7932) (-64.0618, -27.26) (-64.0618, -27.7034) knots 0 0 0 1 2 2 2
  line L181 (-64.0618, -27.7034) -> (-64.0618, -29.2619)
  line L182 (-61.6086, -29.2619) -> (-62.0131, -29.2619)
  line L183 (-62.0131, -29.2619) -> (-62.0131, -27.8927)
  spline S232 degree 2 poles (-62.0131, -27.8927) (-62.0131, -27.7267) (-62.0442, -27.4415) (-62.0909, -27.3559) knots 0 0 0 1 2 2 2
  spline S233 degree 2 poles (-62.0909, -27.3559) (-62.1402, -27.2651) (-62.3165, -27.177) (-62.4669, -27.177) knots 0 0 0 1 2 2 2
  spline S234 degree 2 poles (-62.4669, -27.177) (-62.6173, -27.177) (-62.9363, -27.3377) (-63.0893, -27.4674) knots 0 0 0 1 2 2 2
  line L184 (-63.0893, -27.4674) -> (-63.0893, -29.2619)
  line L185 (-63.0893, -29.2619) -> (-63.4938, -29.2619)
  line L186 (-63.4938, -29.2619) -> (-63.4938, -26.8606)
  line L187 (-63.4938, -26.8606) -> (-63.0893, -26.8606)
  line L188 (-63.0893, -26.8606) -> (-63.0893, -27.1277)
  spline S235 degree 2 poles (-63.0893, -27.1277) (-62.9078, -26.9643) (-62.5577, -26.7932) (-62.3606, -26.7932) knots 0 0 0 1 2 2 2
  spline S236 degree 2 poles (-62.3606, -26.7932) (-62.0079, -26.7932) (-61.6086, -27.26) (-61.6086, -27.7034) knots 0 0 0 1 2 2 2
  line L189 (-61.6086, -27.7034) -> (-61.6086, -29.2619)
  line L190 (-57.781, -29.2619) -> (-59.6352, -29.2619)
  line L191 (-59.6352, -29.2619) -> (-59.6352, -26.0619)
  line L192 (-59.6352, -26.0619) -> (-59.2099, -26.0619)
  line L193 (-59.2099, -26.0619) -> (-59.2099, -28.8833)
  line L194 (-59.2099, -28.8833) -> (-57.781, -28.8833)
  line L195 (-57.781, -28.8833) -> (-57.781, -29.2619)
  spline S237 degree 2 poles (-56.1395, -29.0078) (-56.1888, -29.0441) (-56.3548, -29.1737) (-56.4326, -29.2126) knots 0 0 0 1 2 2 2
  spline S238 degree 2 poles (-56.4326, -29.2126) (-56.5389, -29.2697) (-56.7386, -29.3293) (-56.9201, -29.3293) knots 0 0 0 1 2 2 2
  spline S239 degree 2 poles (-56.9201, -29.3293) (-57.0679, -29.3293) (-57.335, -29.2178) (-57.4361, -29.1167) knots 0 0 0 1 2 2 2
  spline S240 degree 2 poles (-57.4361, -29.1167) (-57.5321, -29.0181) (-57.6488, -28.7277) (-57.6488, -28.5669) knots 0 0 0 1 2 2 2
  spline S241 degree 2 poles (-57.6488, -28.5669) (-57.6488, -28.318) (-57.4387, -27.9653) (-57.2105, -27.8642) knots 0 0 0 1 2 2 2
  spline S242 degree 2 poles (-57.2105, -27.8642) (-57.0083, -27.7708) (-56.4585, -27.7008) (-56.1395, -27.6826) knots 0 0 0 1 2 2 2
  line L196 (-56.1395, -27.6826) -> (-56.1395, -27.6048)
  spline S243 degree 2 poles (-56.1395, -27.6048) (-56.1395, -27.4648) (-56.2251, -27.2911) (-56.3029, -27.2418) knots 0 0 0 1 2 2 2
  spline S244 degree 2 poles (-56.3029, -27.2418) (-56.3807, -27.1925) (-56.6037, -27.1614) (-56.723, -27.1614) knots 0 0 0 1 2 2 2
  spline S245 degree 2 poles (-56.723, -27.1614) (-56.863, -27.1614) (-57.2417, -27.2444) (-57.431, -27.3248) knots 0 0 0 1 2 2 2
  line L197 (-57.431, -27.3248) -> (-57.4543, -27.3248)
  line L198 (-57.4543, -27.3248) -> (-57.4543, -26.9125)
  spline S246 degree 2 poles (-57.4543, -26.9125) (-57.3428, -26.8813) (-56.9253, -26.8035) (-56.7204, -26.8035) knots 0 0 0 1 2 2 2
  spline S247 degree 2 poles (-56.7204, -26.8035) (-56.4715, -26.8035) (-56.1318, -26.8813) (-55.9969, -26.9825) knots 0 0 0 1 2 2 2
  spline S248 degree 2 poles (-55.9969, -26.9825) (-55.8647, -27.081) (-55.735, -27.3948) (-55.735, -27.6204) knots 0 0 0 1 2 2 2
  line L199 (-55.735, -27.6204) -> (-55.735, -29.2619)
  line L200 (-55.735, -29.2619) -> (-56.1395, -29.2619)
  line L201 (-56.1395, -29.2619) -> (-56.1395, -29.0078)
  line L202 (-56.1395, -28.6706) -> (-56.1395, -28.0042)
  spline S249 degree 2 poles (-56.1395, -28.0042) (-56.2848, -28.0172) (-56.723, -28.0612) (-56.8605, -28.1027) knots 0 0 0 1 2 2 2
  spline S250 degree 2 poles (-56.8605, -28.1027) (-57.0212, -28.152) (-57.2313, -28.3569) (-57.2313, -28.5384) knots 0 0 0 1 2 2 2
  spline S251 degree 2 poles (-57.2313, -28.5384) (-57.2313, -28.7459) (-56.9979, -28.9559) (-56.7749, -28.9559) knots 0 0 0 1 2 2 2
  spline S252 degree 2 poles (-56.7749, -28.9559) (-56.5856, -28.9559) (-56.2744, -28.7925) (-56.1395, -28.6706) knots 0 0 0 1 2 2 2
  line L203 (-52.4442, -29.2619) -> (-52.4442, -27.8719)
  spline S253 degree 2 poles (-52.4442, -27.8719) (-52.4442, -27.706) (-52.4702, -27.4233) (-52.5117, -27.3455) knots 0 0 0 1 2 2 2
  spline S254 degree 2 poles (-52.5117, -27.3455) (-52.5532, -27.26) (-52.7113, -27.177) (-52.8488, -27.177) knots 0 0 0 1 2 2 2
  spline S255 degree 2 poles (-52.8488, -27.177) (-52.9733, -27.177) (-53.2585, -27.33) (-53.4089, -27.4752) knots 0 0 0 1 2 2 2
  spline S256 degree 2 poles (-53.4089, -27.4752) (-53.4063, -27.5115) (-53.4011, -27.6126) (-53.4011, -27.68) knots 0 0 0 1 2 2 2
  line L204 (-53.4011, -27.68) -> (-53.4011, -29.2619)
  line L205 (-53.4011, -29.2619) -> (-53.8057, -29.2619)
  line L206 (-53.8057, -29.2619) -> (-53.8057, -27.8719)
  spline S257 degree 2 poles (-53.8057, -27.8719) (-53.8057, -27.706) (-53.8316, -27.4233) (-53.8731, -27.3455) knots 0 0 0 1 2 2 2
  spline S258 degree 2 poles (-53.8731, -27.3455) (-53.9146, -27.26) (-54.0728, -27.177) (-54.2102, -27.177) knots 0 0 0 1 2 2 2
  spline S259 degree 2 poles (-54.2102, -27.177) (-54.3399, -27.177) (-54.6277, -27.3403) (-54.7626, -27.4674) knots 0 0 0 1 2 2 2
  line L207 (-54.7626, -27.4674) -> (-54.7626, -29.2619)
  line L208 (-54.7626, -29.2619) -> (-55.1671, -29.2619)
  line L209 (-55.1671, -29.2619) -> (-55.1671, -26.8606)
  line L210 (-55.1671, -26.8606) -> (-54.7626, -26.8606)
  line L211 (-54.7626, -26.8606) -> (-54.7626, -27.1251)
  spline S260 degree 2 poles (-54.7626, -27.1251) (-54.6044, -26.9669) (-54.2932, -26.7932) (-54.1065, -26.7932) knots 0 0 0 1 2 2 2
  spline S261 degree 2 poles (-54.1065, -26.7932) (-53.8938, -26.7932) (-53.5645, -26.9877) (-53.4789, -27.2081) knots 0 0 0 1 2 2 2
  spline S262 degree 2 poles (-53.4789, -27.2081) (-53.2948, -27.0032) (-52.9473, -26.7932) (-52.7451, -26.7932) knots 0 0 0 1 2 2 2
  spline S263 degree 2 poles (-52.7451, -26.7932) (-52.5895, -26.7932) (-52.3353, -26.8891) (-52.242, -26.998) knots 0 0 0 1 2 2 2
  spline S264 degree 2 poles (-52.242, -26.998) (-52.146, -27.107) (-52.0397, -27.4337) (-52.0397, -27.68) knots 0 0 0 1 2 2 2
  line L212 (-52.0397, -27.68) -> (-52.0397, -29.2619)
  line L213 (-52.0397, -29.2619) -> (-52.4442, -29.2619)
  spline S265 degree 2 poles (-49.4595, -28.0223) (-49.4595, -28.611) (-50.03, -29.3293) (-50.4605, -29.3293) knots 0 0 0 1 2 2 2
  spline S266 degree 2 poles (-50.4605, -29.3293) (-50.6549, -29.3293) (-50.9324, -29.2334) (-51.0673, -29.1504) knots 0 0 0 1 2 2 2
  line L214 (-51.0673, -29.1504) -> (-51.0932, -29.2619)
  line L215 (-51.0932, -29.2619) -> (-51.4718, -29.2619)
  line L216 (-51.4718, -29.2619) -> (-51.4718, -25.9193)
  line L217 (-51.4718, -25.9193) -> (-51.0673, -25.9193)
  line L218 (-51.0673, -25.9193) -> (-51.0673, -27.1121)
  spline S267 degree 2 poles (-51.0673, -27.1121) (-50.9143, -26.9747) (-50.559, -26.7932) (-50.3334, -26.7932) knots 0 0 0 1 2 2 2
  spline S268 degree 2 poles (-50.3334, -26.7932) (-49.9263, -26.7932) (-49.4595, -27.4441) (-49.4595, -28.0223) knots 0 0 0 1 2 2 2
  spline S269 degree 2 poles (-49.877, -28.0535) (-49.877, -27.623) (-50.1389, -27.177) (-50.4293, -27.177) knots 0 0 0 1 2 2 2
  spline S270 degree 2 poles (-50.4293, -27.177) (-50.5927, -27.177) (-50.9298, -27.3326) (-51.0673, -27.4518) knots 0 0 0 1 2 2 2
  line L219 (-51.0673, -27.4518) -> (-51.0673, -28.8288)
  spline S271 degree 2 poles (-51.0673, -28.8288) (-50.9143, -28.904) (-50.6783, -28.9663) (-50.5383, -28.9663) knots 0 0 0 1 2 2 2
  spline S272 degree 2 poles (-50.5383, -28.9663) (-50.2297, -28.9663) (-49.877, -28.528) (-49.877, -28.0535) knots 0 0 0 1 2 2 2
  spline S273 degree 2 poles (-47.9969, -29.3164) (-48.5726, -29.3164) (-49.2053, -28.6706) (-49.2053, -28.0742) knots 0 0 0 1 2 2 2
  spline S274 degree 2 poles (-49.2053, -28.0742) (-49.2053, -27.4882) (-48.5908, -26.7932) (-48.0955, -26.7932) knots 0 0 0 1 2 2 2
  spline S275 degree 2 poles (-48.0955, -26.7932) (-47.8724, -26.7932) (-47.5276, -26.9228) (-47.4005, -27.0603) knots 0 0 0 1 2 2 2
  spline S276 degree 2 poles (-47.4005, -27.0603) (-47.2708, -27.1977) (-47.1334, -27.5945) (-47.1334, -27.8823) knots 0 0 0 1 2 2 2
  line L220 (-47.1334, -27.8823) -> (-47.1334, -28.1027)